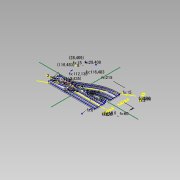
# Autodesk Inventor part: SingleCross
Saved by Autodesk Inventor 2021 (Build 250183000, 183)
## iProperties
Created: 2021-03-17
Part Number: SingleCross
Material: 一般
Document SubType Name: Modeling
Designer: kumagai
Density: 1 g/cm^3
Appearance: 既定
d2: 18.600 mm
d3: 2.400 mm
d4: 2.000 mm
d5: 38.000 mm
d6: 60.000 mm
d7: 30.00 deg
d8: 38.000 mm
d9: 18.600 mm
d10: 2.000 mm
d11: 2.400 mm
d12: 215.000 mm
d13: 15.000 mm
d14: 15.000 mm
d27: 10.00 deg
d28: 15.00 deg
d29: 3.000 mm
d32: 2.500 mm
d33: 1.500 mm
d34: 1.000 mm
d35: 10.00 deg
d36: 15.00 deg
d37: 3.000 mm
d39: 10.00 deg
d40: 15.00 deg
d41: 3.000 mm
d45: 2.800 mm
d46: 2.500 mm
d47: 1.000 mm
d51: 8.000 mm
d52: 8.000 mm
d55: 8.500 mm
d56: 2.400 mm
d57: 2.400 mm
d58: 1.000 mm
d61: 59.245 mm
d62: 8.000 mm
d64: 3.000 mm
d68: 3.000 mm
d69: 1.000 mm
d73: 28.409 mm
d74: 116.483 mm
d75: 112.135 mm
d76: 1.000 mm
d78: 5.000 mm
d80: 2.100 mm
d81: 1.000 mm
d83: 6.000 mm
d84: 3.200 mm
d85: 0.00 deg
d86: 5.200 mm
d87: 0.00 deg
d54: 112.135 mm
d59: 112.135 mm
d60: 59.245 mm
d71: 28.409 mm
d72: 116.483 mm
PrinterOffset: 0.000 mm
StraightLength: 215.000 mm
RailWidth: 38.000 mm
OuterWall: 2.000 mm
InnerWall: 2.400 mm
InsideWidth: 18.600 mm
RailHeight: 8.400 mm
RailDepth: 3.200 mm
ConnectorLength: 15.000 mm
JointMW1: 13.000 mm
JointMW2: 9.400 mm
JointMH: 9.000 mm
JointFW1: 13.300 mm
JointFW2: 9.600 mm
JointFH: 9.500 mm
DoubleWidth: 60.000 mm
ViaductHeight: 66.000 mm
SupportGap: 0.200 mm
SupportRib: 0.500 mm
BarCX: 28.409 mm
BarCY: 116.483 mm
BarL: 59.245 mm
BarR: 112.135 mm
Author: kumagai
Autodesk Inventor part; units mm, degrees
ref_plane "YZ Plane" through (0, 0, 0) normal (1, 0, 0) x (0, 1, 0)
ref_plane "XZ Plane" through (0, 0, 0) normal (0, 1, 0) x (-1, 0, 0)
ref_plane "XY Plane" through (0, 0, 0) normal (0, 0, 1) x (1, 0, 0)
sketch "スケッチ1" plane through (0, 0, 0) normal (0, 1, 0) x (-1, 0, 0)
  line L0 (0, -142.4661) -> (0, 130.4188) projected
  line L1 (-213.4501, 0) -> (176.9459, 0) projected
  line L2 (92.5, -64.2765) -> (92.5, -56.9696)
  line L3 (-92.5, -64.2765) -> (-92.5, -56.9696)
  line L4 (-117.7076, 30) -> (-128.5713, 30)
  line L5 (-121.2644, 36.9) -> (-128.5713, 36.9)
  line L6 (-121.2644, 39.3) -> (-128.5713, 39.3)
  line L7 (-121.2644, 47) -> (-128.5713, 47)
  line L8 (-121.2644, 49) -> (-128.5713, 49)
  line L9 (-121.2644, 23.1) -> (-128.5713, 23.1)
  line L10 (-121.2644, 20.7) -> (-128.5713, 20.7)
  line L11 (-121.2644, 13) -> (-128.5713, 13)
  line L12 (-121.2644, 11) -> (-128.5713, 11)
  line L13 (-117.7076, -30) -> (-128.5713, -30)
  line L14 (-121.2644, -36.9) -> (-128.5713, -36.9)
  line L15 (-121.2644, -39.3) -> (-128.5713, -39.3)
  line L16 (-121.2644, -47) -> (-128.5713, -47)
  line L17 (-121.2644, -49) -> (-128.5713, -49)
  line L18 (-121.2644, -23.1) -> (-128.5713, -23.1)
  line L19 (-121.2644, -20.7) -> (-128.5713, -20.7)
  line L20 (-121.2644, -13) -> (-128.5713, -13)
  line L21 (-121.2644, -11) -> (-128.5713, -11)
  line L22 (-112.5706, 30) -> (121.1751, 30)
  line L23 (-129.3491, -74.6797) -> (118.7156, 68.5405)
  line L24 (-145.7027, -76.1541) -> (-152.6826, -80.1839)
  line L25 (-145.8493, -73.4674) -> (-152.8292, -77.4973)
  line L26 (-149.6993, -66.799) -> (-156.6792, -70.8289)
  line L27 (-150.6993, -65.067) -> (-157.6792, -69.0968)
  line L28 (-128.5713, -49) -> (-128.5713, -11)
  line L29 (-128.5713, 11) -> (-128.5713, 49)
  line L30 (-157.6792, -69.0968) -> (-138.6792, -102.0058)
  line L31 (-138.8027, -88.1052) -> (-145.7826, -92.135)
  line L32 (-136.5493, -89.5755) -> (-143.5292, -93.6053)
  line L33 (-132.6993, -96.2439) -> (-139.6792, -100.2737)
  line L34 (-131.6993, -97.976) -> (-138.6792, -102.0058)
  line L35 (-92.5, 49) -> (92.5, 49)
  line L36 (-92.5, -49) -> (-84.5, -49)
  line L37 (-92.5, -49) -> (-92.5, -11)
  line L38 (-92.5, -11) -> (-84.5, -11)
  line L39 (-92.5, -13) -> (-84.5, -13)
  line L40 (-92.5, -20.7) -> (-84.5, -20.7)
  line L41 (-92.5, -23.1) -> (-84.5, -23.1)
  line L42 (-92.5, -36.9) -> (-84.5, -36.9)
  line L43 (-92.5, -39.3) -> (-84.5, -39.3)
  line L44 (-92.5, -47) -> (-84.5, -47)
  line L45 (-92.5, 47) -> (92.5, 47)
  line L46 (92.5, 36.9) -> (84.5, 36.9)
  line L47 (-92.5, 20.7) -> (0.4065, 20.7)
  line L48 (92.5, 13) -> (89.5, 13)
  line L49 (92.5, 11) -> (92.5, 49)
  line L50 (-92.5, 11) -> (-92.5, 49)
  line L51 (107.5, -64.2765) -> (107.5, -56.9696)
  line L52 (-107.5, -64.2765) -> (-107.5, -56.9696)
  line L53 (20.6487, 3.9541) -> (-20.3324, -19.7063)
  line L54 (23.8097, 3.0078) -> (-19.1324, -21.7848)
  line L55 (32.2824, -0.9917) -> (-15.2824, -28.4532)
  line L56 (33.2824, -2.7237) -> (-14.2824, -30.1852)
  line L57 (5.2526, 11) -> (-27.2324, -7.7552)
  line L58 (3.9167, 13) -> (-28.4324, -5.6767)
  arc A0 (-84.5, -11) -> (-33.2824, 2.7237) centre (-84.5, 91.4352) ccw
  arc A1 (-84.5, -13) -> (-32.2824, 0.9917) centre (-84.5, 91.4352) ccw
  arc A2 (-84.5, -20.7) -> (-28.4324, -5.6767) centre (-84.5, 91.4352) ccw
  arc A3 (-84.5, -23.1) -> (-27.2324, -7.7552) centre (-84.5, 91.4352) ccw
  arc A4 (-84.5, -36.9) -> (-20.3324, -19.7063) centre (-84.5, 91.4352) ccw
  arc A5 (-84.5, -39.3) -> (-19.1324, -21.7848) centre (-84.5, 91.4352) ccw
  arc A6 (-84.5, -47) -> (-15.2824, -28.4532) centre (-84.5, 91.4352) ccw
  arc A7 (-84.5, -49) -> (-14.2824, -30.1852) centre (-84.5, 91.4352) ccw
  line L59 (89.5, 11) -> (92.5, 11)
  line L60 (84.5, 39.3) -> (92.5, 39.3)
  arc A8 (54.2413, 6.4289) -> (33.2824, -2.7237) centre (84.5, -91.4352) ccw
  arc A9 (53.6505, 8.3397) -> (32.2824, -0.9917) centre (84.5, -91.4352) ccw
  line L61 (21.1323, 13) -> (3.9167, 13)
  line L62 (5.2526, 11) -> (18.9976, 11)
  line L63 (0.4065, 23.1) -> (-92.5, 23.1)
  line L64 (-25.8095, 4.7288) -> (-32.2824, 0.9917)
  line L65 (-26.8095, 6.4608) -> (-33.2824, 2.7237)
  line L66 (-92.5, 11) -> (-28.8019, 11)
  line L67 (-23.0422, 9.5625) -> (-28.0254, 10.8978)
  line L68 (-26.3812, 6.7608) -> (-23.0422, 9.5625)
  line L69 (-28.8019, 13) -> (-92.5, 13)
  line L70 (-25.0956, 5.2287) -> (-20.285, 9.2652)
  line L71 (-27.5078, 12.8296) -> (-20.669, 10.9972)
  arc A10 (-26.8095, 6.4608) -> (-26.3812, 6.7608) centre (-28.3095, 9.0589) ccw
  arc A11 (-28.0254, 10.8978) -> (-28.8019, 11) centre (-28.8019, 8) ccw
  arc A12 (-27.5078, 12.8296) -> (-28.8019, 13) centre (-28.8019, 8) ccw
  arc A13 (-25.8095, 4.7288) -> (-25.0956, 5.2287) centre (-28.3095, 9.0589) ccw
  arc A14 (-20.285, 9.2652) -> (-20.669, 10.9972) centre (-20.9278, 10.0313) ccw
  arc A15 (0.4065, 23.1) -> (1.9065, 23.5019) centre (0.4065, 26.1) ccw
  arc A16 (0.4065, 20.7) -> (3.1065, 21.4235) centre (0.4065, 26.1) ccw
  line L72 (3.1065, 21.4235) -> (11.3782, 26.1991)
  line L73 (1.9065, 23.5019) -> (10.1782, 28.2776)
  line L74 (14.0984, 36.9) -> (-92.5, 36.9)
  line L75 (15.496, 39.116) -> (22.2839, 37.2972)
  line L76 (12.1493, 26.739) -> (22.6679, 35.5652)
  line L77 (10.6066, 28.5775) -> (19.065, 35.675)
  line L78 (-92.5, 39.3) -> (14.0984, 39.3)
  line L79 (19.065, 35.675) -> (14.8749, 36.7978)
  arc A17 (10.1782, 28.2776) -> (10.6066, 28.5775) centre (8.6782, 30.8757) ccw
  arc A18 (11.3782, 26.1991) -> (12.1493, 26.739) centre (8.6782, 30.8757) ccw
  arc A19 (15.496, 39.116) -> (14.0984, 39.3) centre (14.0984, 33.9) ccw
  arc A20 (14.8749, 36.7978) -> (14.0984, 36.9) centre (14.0984, 33.9) ccw
  arc A21 (22.6679, 35.5652) -> (22.2839, 37.2972) centre (22.0251, 36.3313) ccw
  arc A22 (84.5, 39.3) -> (20.5153, 22.572) centre (84.5, -91.4352) ccw
  line L80 (84.5, -31.1736) -> (84.5, -39.0158)
  line L81 (-84.5, 55.9571) -> (-84.5, 64.7286)
  arc A23 (21.9177, 11.381) -> (23.6803, 4.8027) centre (25.2554, 8.75) ccw
  arc A24 (18.9976, 11) -> (20.6487, 3.9541) centre (25.2554, 8.75) ccw
  arc A25 (23.8097, 3.0078) -> (23.6803, 4.8027) centre (23.3097, 3.8739) ccw
  arc A26 (21.9177, 11.381) -> (21.1323, 13) centre (21.1323, 12) ccw
  arc A27 (65.4055, 19.0623) -> (31.4293, 7.3464) centre (84.5, -91.4352) ccw
  line L82 (82.3191, 24.681) -> (81.5639, 27.454)
  line L83 (80.3363, 28.1561) -> (53.2692, 20.7843)
  line L84 (84.6348, 25.3117) -> (83.8795, 28.0847)
  line L85 (79.7056, 30.4717) -> (52.6385, 23.1)
  line L86 (84.5, 8) -> (84.5, 6.2824)
  line L87 (86.5, 8) -> (86.5, 6.2824)
  line L88 (21.0047, 20.7) -> (52.6385, 20.7)
  line L89 (87.5293, 20.7) -> (92.5, 20.7)
  arc A28 (52.6385, 20.7) -> (53.2692, 20.7843) centre (52.6385, 23.1) ccw
  line L90 (92.5, 23.1) -> (87.5293, 23.1)
  line L91 (52.6385, 23.1) -> (26.6069, 23.1)
  arc A29 (89.5, 11) -> (86.5, 8) centre (89.5, 8) ccw
  arc A30 (89.5, 13) -> (84.5, 8) centre (89.5, 8) ccw
  arc A31 (82.3191, 24.681) -> (87.5293, 20.7) centre (87.5293, 26.1) ccw
  arc A32 (84.6348, 25.3117) -> (87.5293, 23.1) centre (87.5293, 26.1) ccw
  arc A33 (81.5639, 27.454) -> (80.3363, 28.1561) centre (80.599, 27.1912) ccw
  arc A34 (83.8795, 28.0847) -> (79.7056, 30.4717) centre (80.599, 27.1912) ccw
  arc A35 (83.2577, 5.3122) -> (55.6934, 8.652) centre (56.0914, -103.4826) ccw
  arc A36 (82.7732, 3.3718) -> (55.7005, 6.652) centre (56.0914, -103.4826) ccw
  arc A37 (83.2577, 5.3122) -> (84.5, 6.2824) centre (83.5, 6.2824) ccw
  arc A38 (82.7732, 3.3718) -> (86.5, 6.2824) centre (83.5, 6.2824) ccw
  arc A39 (55.7005, 6.652) -> (54.2413, 6.4289) centre (55.7183, 1.652) ccw
  arc A40 (55.6934, 8.652) -> (53.6505, 8.3397) centre (55.7183, 1.652) ccw
  circle A41 centre (25.2554, 8.75) radius 1.05
  arc A42 (84.5, 36.9) -> (26.6069, 23.1) centre (84.5, -91.4352) ccw
  arc A43 (20.5153, 22.572) -> (21.0047, 20.7) centre (21.0047, 21.7) ccw
  line L92 (-80.5, 11) -> (-86.5, 11)
  line L93 (-86.5, 7) -> (-86.5, 0)
  line L94 (-86.5, 0) -> (-80.5, 0)
  line L95 (-80.5, 0) -> (-80.5, 7)
  arc A44 (-76.5, 11) -> (-80.5, 7) centre (-76.5, 7) ccw
  arc A45 (-86.5, 7) -> (-90.5, 11) centre (-90.5, 7) ccw
  point P0 (0, 0)
  point P1 (-63.9127, -36.9)
  point P2 (25.2554, 13)
  point P3 (-18.8135, 10.5)
  point P4 (24.1395, 36.8)
  point P5 (27.3804, 5.0694)
  point P6 (83.4033, 20.7)
  point P7 (84.5, 4.9945)
  point P8 (82.5149, 30)
  point P9 (77.9735, 30)
  point P10 (-86.5, 11)
  point P11 (-80.5, 0)
  dimension "JointMW1" = 13
  dimension "d2" = 18.6
  dimension "d3" = 2.4
  dimension "d4" = 2
  dimension "d5" = 38
  dimension "d6" = 60
  dimension "d7" = 30
  dimension "d8" = 38
  dimension "d9" = 18.6
  dimension "d10" = 2
  dimension "d11" = 2.4
  dimension "d12" = 215
  dimension "d13" = 15
  dimension "d14" = 15
  dimension "d29" = 3
  dimension "d32" = 2.5
  dimension "d33" = 1.5
  dimension "d34" = 1
  dimension "d35" = 10
  dimension "d36" = 15
  dimension "d37" = 3
  dimension "d39" = 10
  dimension "d40" = 15
  dimension "d41" = 3
  dimension "d45" = 2.8
  dimension "d46" = 2.5
  dimension "d47" = 1
  dimension "d51" = 8
  dimension "d52" = 8
  dimension "d54" = 112.1352
  dimension "d55" = 8.5
  dimension "d57" = 2.4
  dimension "d58" = 1
  dimension "d59" = 112.1352
  dimension "d60" = 59.2446
  dimension "d61" = 59.2446
  dimension "d62" = 8
  dimension "d64" = 3
  dimension "d68" = 3
  dimension "d69" = 1
  dimension "d71" = 28.4086
  dimension "d72" = 116.4826
  dimension "d73" = 28.4086
  dimension "d74" = 116.4826
  dimension "d75" = 112.1352
  dimension "d76" = 1
  dimension "d78" = 5
  dimension "d80" = 2.1
  dimension "d81" = 1
  dimension "d83" = 6
  dimension "d88" = 4
  constraints: 188 end point, 93 point on circle, 86 tangent, 46 centre point, 42 point on line, 41 collinear, 34 symmetric about line, 29 horizontal, 22 parallel, 21 coincident, 11 vertical, 8 equal length, 4 equal radius, 4 perpendicular, 4 vertical alignment, 3 horizontal alignment, 2 other
  measures "d2" distance between parallel lines of L6 L10
  measures "d3" distance between parallel lines of L6 L5
  measures "d4" distance between parallel lines of L8 L7
  measures "d5" distance between parallel lines of L8 L12
  measures "d6" distance between parallel lines of L4 L13
  measures "d7" angle of L23 L1
  measures "d8" distance between parallel lines of L27 L34
  measures "d9" distance between parallel lines of L25 L32
  measures "d10" distance between parallel lines of L27 L26
  measures "d11" distance between parallel lines of L25 L24
  measures "d12" distance between parallel lines of L52 L51
  measures "d13" distance between parallel lines of L51 L2
  measures "d14" distance between parallel lines of L3 L52
  measures "d29" radius of A10
  measures "d32" distance from line of point (-18.813, 10.5) L69
  measures "d33" distance from line of point (-18.813, 10.5) L64
  measures "d34" radius of A14
  measures "d35" angle of L64 L70
  measures "d36" angle of L69 L71
  measures "d37" radius of A15
  measures "d39" angle of L72 L76
  measures "d40" angle of L78 L75
  measures "d41" radius of A17
  measures "d45" distance from line of point (24.139, 36.8) L72
  measures "d46" distance from line of point (24.139, 36.8) L78
  measures "d47" radius of A21
  measures "d51" distance between parallel lines of L80 L2
  measures "d52" distance between parallel lines of L81 L3
  measures "d54" radius of A2
  measures "d55" diameter of A23
  measures "d57" radial gap between concentric circles of A24 A23
  measures "d58" radius of A25
  measures "d59" radius of A27
  measures "d60" distance from line of L86 A23.centre
  measures "d61" distance from line of L82 A23.centre
  measures "d62" distance from line of point (83.403, 20.7) L83
  measures "d64" radius of A29
  measures "d68" radius of A32
  measures "d69" radius of A33
  measures "d71" distance from line of A22.centre L82
  measures "d72" distance from line of A22.centre L83
  measures "d73" distance from line of A35.centre L86
  measures "d74" distance from line of A35.centre L48
  measures "d75" radius of A35
  measures "d76" radius of A37
  measures "d78" radius of A39
  measures "d80" diameter of A41
  measures "d81" radius of A43
  measures "d83" distance between parallel lines of L95 L93
  measures "d88" radius of A44
extrude "押し出し1" add sketch "スケッチ1" along normal blind 3.2 contours L56 A7 L36 L23 A6 L55 L0 | L0 L55 A9 L1 A8 L56 | L54 A5 L23 A4 L53 L0 | L0 L53 L1 L54 | L1 A9 A40 A35 A37 L86 A30 L48 L49 L59 A29 L87 A38 A36 A39 A8 | L1 L53 A24 L23 A26 A23 A25 L54 | L23 L36 L37 L44 A6 | A5 L43 L37 L42 A4 L23 | L57 L1 L58 L0 | L0 L58 L61 A26 L23 A24 L62 L57 | L57 A3 L41 L37 L40 A2 L58 L1 | L47 L50 L63 L0 | L0 L63 A15 L73 A17 L77 L22 L76 A18 L72 A16 L47 | A1 L39 L37 L38 A0 L1 | L1 A0 L65 A10 L68 L67 A11 L66 L50 L69 A12 L71 A14 L70 A13 L64 A1 | L88 A43 A22 L22 A42 L91 L23 | L23 L91 L85 L22 A34 L84 A32 L90 L49 L89 A31 L82 A33 L83 A28 L88 | L74 L50 L78 L0 | L0 L78 A19 L75 A21 L76 L22 L77 L79 A20 L74 | L22 A22 L23 A42 | L23 A22 L60 L49 L46 A42 | L45 L50 L35 L0 | L0 L35 L23 L45 | L23 L35 L49 L45
extrude "押し出し2" add sketch "スケッチ1" against normal blind 5.2 contours L56 A7 L36 L23 A6 L55 L0 | L0 L55 A9 L1 A8 L56 | L55 A6 L23 A5 L54 L0 | L0 L54 L1 A9 L55 | L54 A5 L23 A4 L53 L0 | L0 L53 L1 L54 | L1 A9 A40 A35 A37 L86 A30 L48 L49 L59 A29 L87 A38 A36 A39 A8 | L53 A4 L23 L0 | L0 L1 L53 | L54 A25 A23 A26 L23 L88 A28 L83 A33 L82 A31 L89 L49 L48 A30 L86 A37 A35 A40 A9 L1 | L1 L53 A24 L23 A26 A23 A25 L54 | A6 L44 L37 L43 A5 L23 | L23 L36 L37 L44 A6 | L1 L57 L0 | L23 A4 L42 L37 L41 A3 L57 L1 | L23 A24 L53 L1 | L0 L57 L62 A24 L23 | A5 L43 L37 L42 A4 L23 | L57 L1 L58 L0 | L0 L58 L61 A26 L23 A24 L62 L57 | L57 A3 L41 L37 L40 A2 L58 L1 | L58 L1 A1 L64 A13 L70 A14 L71 A12 L69 L50 L47 L0 | L0 L47 A16 L72 A18 L76 L22 A22 A43 L88 L23 A26 L61 L58 | L58 A2 L40 L37 L39 A1 L1 | L47 L50 L63 L0 | L0 L63 A15 L73 A17 L77 L22 L76 A18 L72 A16 L47 | A1 L39 L37 L38 A0 L1 | L1 A0 L65 A10 L68 L67 A11 L66 L50 L69 A12 L71 A14 L70 A13 L64 A1 | L88 A43 A22 L22 A42 L91 L23 | L23 L91 L85 L22 A34 L84 A32 L90 L49 L89 A31 L82 A33 L83 A28 L88 | L63 L50 L22 L0 | L0 L22 L77 A17 L73 A15 L63 | L91 A42 L22 L23 | L23 L22 L85 L91 | L22 L50 L74 L0 | L0 L74 A20 L79 L77 L22 | L1 L93 A45 L66 A44 L95 | L23 A42 L46 L49 L22 A34 L85 | L22 A42 L23 | L74 L50 L78 L0 | L0 L78 A19 L75 A21 L76 L22 L77 L79 A20 L74 | L22 A22 L23 A42 | L85 A34 L22 | L23 A22 L60 L49 L46 A42 | L22 L76 A21 L75 A19 L78 L0 L45 L23 A22 | L78 L50 L45 L0 | L22 L49 L90 A32 L84 A34 | L23 L45 L49 L60 A22 | L45 L50 L35 L0 | L0 L35 L23 L45 | L23 L35 L49 L45
sketch "スケッチ2" plane through (0, -5.2, 0) normal (0, -1, 0) x (1, 0, 0)
  circle A0 centre (-25.2554, 8.75) radius 1.05 projected
  line L0 (-25.2554, 6.3829) -> (-27.3054, 7.5664)
  line L1 (-27.3054, 7.5664) -> (-27.3054, 9.9336)
  line L2 (-27.3054, 9.9336) -> (-25.2554, 11.1171)
  line L3 (-25.2554, 11.1171) -> (-23.2054, 9.9336)
  line L4 (-23.2054, 9.9336) -> (-23.2054, 7.5664)
  line L5 (-23.2054, 7.5664) -> (-25.2554, 6.3829)
  point P0 (0, 0)
  dimension "d89" = 4.1
  constraints: 12 end point, 1 coincident, 1 vertical, 13 other
  measures "d89" distance between parallel lines of L1 L4
extrude "押し出し3" cut sketch "スケッチ2" against normal blind 2.5 contours A0 | L0 L1 L2 L3 L4 L5
equation "\"d2\" = InsideWidth"
equation "\"d3\" = InnerWall"
equation "\"d4\" = OuterWall"
equation "\"d5\" = RailWidth"
equation "\"d6\" = DoubleWidth"
equation "\"d8\" = RailWidth"
equation "\"d9\" = InsideWidth"
equation "\"d10\" = OuterWall"
equation "\"d11\" = InnerWall"
equation "\"d12\" = StraightLength"
equation "\"d13\" = ConnectorLength"
equation "\"d14\" = ConnectorLength"
equation "\"BarCX\" = 28.40864"
equation "\"BarCY\" = 116.48256"
equation "\"BarR\" = 112.13524"
equation "\"BarL\" = 59.24456"
equation "\"InsideWidth\" = 18.6"
equation "\"InnerWall\" = 2.4"
equation "\"OuterWall\" = 2"
equation "\"RailWidth\" = 38"
equation "\"DoubleWidth\" = 60"
equation "\"StraightLength\" = 215"
equation "\"ConnectorLength\" = 15"
